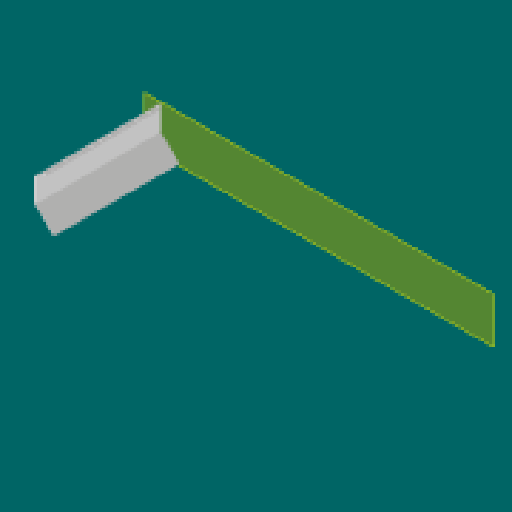
# Autodesk Inventor part: P_PRZ
Saved by Autodesk Inventor 2023 (Build 270158000, 158)
## iProperties
Created: 2023-01-28
Part Number: P_PRZ
Material: Generic
Document SubType Name: Sheet Metal
Designer: HeavyDrewno
Density: 1 g/cm^3
Sheet Metal Rule: Default
Appearance: Default
Author: HeavyDrewno
Autodesk Inventor part; units mm, degrees
ref_plane "YZ Plane" through (0, 0, 0) normal (1, 0, 0) x (0, 1, 0)
ref_plane "XZ Plane" through (0, 0, 0) normal (0, 1, 0) x (-1, 0, 0)
ref_plane "XY Plane" through (0, 0, 0) normal (0, 0, 1) x (1, 0, 0)
ref_plane "Work Plane1" through (0, 0, 0) normal (0, 0, 1) x (1, 0, 0)
sketch "Sketch1" plane through (0, 0, 0) normal (0, 0, 1) x (1, 0, 0)
  line L0 (-508.0208, 63.6072) -> (-508.0208, -12.3928) construction
  line L1 (-508.0208, -12.3928) -> (-450.0898, -68.3928) construction
  spline S0 degree 3 poles (-448.0208, -70.3928) (-448.1361, -70.2662) (-448.309, -70.0762) (-448.8272, -69.5583) (-448.9219, -69.465) (-449.3425, -69.0576) (-449.7132, -68.7169) (-450.0898, -68.3928) knots 0 0 0 0 0.533816 0.533816 0.643932 0.643932 1 1 1 1 construction
  line L2 (-448.0208, -70.3928) -> (-508.0208, -12.3928)
  line L3 (-508.0208, 63.6072) -> (-508.0208, 65.6072) construction
  line L4 (-508.0208, -12.3928) -> (-508.0208, 65.6072)
  point P0 (0, 0)
contour flange "Contour Flange1" sketch "Sketch1" thickness 2 bend radius 2 width 396 along (0, 0, 1) mid plane no both sides no wall seen from (-478.0208, -41.3928, 0) lies toward (0.6950221, 0.7189884, 0) curves L2 L4
bend "Bend1"
corner "Corner1"
fillet "Corner Round1" radius 3 2 edges at (-507.0208, 65.6072, 0) (-507.0208, 65.6072, 396)
sketch "Sketch2" plane through (-506.0208, 65.6072, 393) normal (0, 1, 0) x (1, 0, 0)
  line L0 (998, 15) -> (-2, 15) construction
  line L1 (998, 375) -> (-2, 375) construction
  line L2 (-2, 375) -> (18, 375)
  line L3 (18, 375) -> (18, 15)
  line L4 (18, 15) -> (-2, 15)
  line L5 (-2, 390) -> (-2, 0)
  line L6 (-2, 15) -> (-2, 375)
  point P0 (506.0208, 393)
  dimension "d12" = 20
  measures "d12" distance of L1.end L2.end
sheet face with bend "Face1" sketch "Sketch2" thickness 2 toward (0, 1, 0) bend radius 2 relief straight relief width 2 relief depth 1
bend "Bend2"
sketch "Sketch3" plane through (-506.0208, 67.6072, 393) normal (0, 1, 0) x (1, 0, 0)
  circle A0 centre (8, 385) radius 4.5 construction
  circle A1 centre (8, 5) radius 4.5 construction
  line L0 (-2, 15) -> (-2, 375) projected
  point P0 (506.0208, 393)
  point P1 (8, 345)
  point P2 (8, 45)
  point P3 (8, 305)
  point P4 (8, 265)
  point P5 (8, 225)
  point P6 (8, 85)
  point P7 (8, 125)
  point P8 (8, 165)
  point P9 (8, 85)
  point P10 (8, 45)
  point P11 (8, 195)
  dimension "d18" = 40
  dimension "d19" = 10
  dimension "d20" = 40
  dimension "d21" = 40
  dimension "d22" = 40
  dimension "d23" = 40
  dimension "d24" = 40
  dimension "d25" = 40
  dimension "d26" = 40
  dimension "d27" = 30
  dimension "d28" = 30
  constraints: 2 coincident
  measures "d18" distance of point (8, 345) A0.centre
  measures "d19" distance from line of L0 point (8, 345)
  measures "d20" distance of point (8, 345) point (8, 305)
  measures "d21" distance of point (8, 265) point (8, 305)
  measures "d22" distance of point (8, 225) point (8, 265)
  measures "d23" distance of A1.centre point (8, 45)
  measures "d24" distance of point (8, 45) point (8, 85)
  measures "d25" distance of point (8, 85) point (8, 125)
  measures "d26" distance of point (8, 125) point (8, 165)
  measures "d27" distance of point (8, 195) point (8, 225)
  measures "d28" distance of point (8, 165) point (8, 195)
hole "Hole1" at (-498.0208, 67.6072, 48) at (-498.0208, 67.6072, 348) at (-498.0208, 67.6072, 88) at (-498.0208, 67.6072, 128) at (-498.0208, 67.6072, 168) at (-498.0208, 67.6072, 308) at (-498.0208, 67.6072, 268) at (-498.0208, 67.6072, 228) at (-498.0208, 67.6072, 198) direction (0, -1, 0) diameter 9 depth 2 tip angle 118
equation "\"d34\" = Thickness"
equation "\"d0\" = Thickness"
equation "\"d1\" = BendReliefWidth"
equation "\"d2\" = BendReliefDepth"
equation "\"d3\" = MinimumRemnant"
equation "\"d4\" = TransitionRadius"
equation "\"d6\" = BendRadius"
equation "\"d8\" = CornerReliefSize"
equation "\"d9\" = GapSize"
equation "\"d10\" = JacobiRadiusSize"
equation "\"d13\" = BendRadius"
equation "\"d14\" = BendReliefWidth"
equation "\"d16\" = MinimumRemnant"
equation "\"d15\" = BendReliefDepth"
equation "\"d17\" = TransitionRadius"
equation "\"BendRadius\" = Thickness"
equation "\"BendReliefWidth\" = Thickness"
equation "\"BendReliefDepth\" = 0.5 * Thickness"
equation "\"CornerReliefSize\" = 4 * Thickness"
equation "\"MinimumRemnant\" = 2 * Thickness"
equation "\"TransitionRadius\" = BendRadius"
equation "\"JacobiRadiusSize\" = BendRadius"
equation "\"GapSize\" = Thickness"
equation "\"Thickness\" = 2"
body "Solid1"
